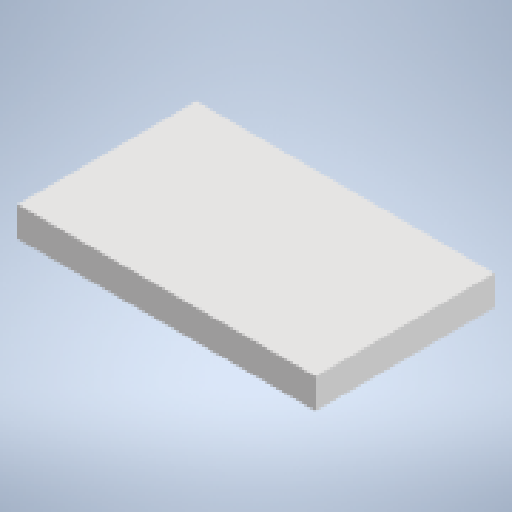
# Autodesk Inventor part: ceiling
Saved by Autodesk Inventor 2024 (Build 280153000, 153)
## iProperties
Created: 2023-05-24
Part Number: ceiling
Material: Generic
Document SubType Name: Modeling
Designer: Patrick
Density: 1 g/cm^3
Appearance: Default
Author: Patrick
Autodesk Inventor part; units mm, degrees
ref_plane "YZ Plane" through (0, 0, 0) normal (1, 0, 0) x (0, 1, 0)
ref_plane "XZ Plane" through (0, 0, 0) normal (0, 1, 0) x (-1, 0, 0)
ref_plane "XY Plane" through (0, 0, 0) normal (0, 0, 1) x (1, 0, 0)
sketch "Sketch1" plane through (0, 0, 0) normal (0, 1, 0) x (-1, 0, 0)
  line L0 (-500, -300) -> (500, -300)
  line L1 (500, -300) -> (500, 300)
  line L2 (500, 300) -> (-500, 300)
  line L3 (-500, 300) -> (-500, -300)
  line L4 (-500, -300) -> (500, 300) construction
  line L5 (500, -300) -> (-500, 300) construction
  point P0 (0, 0)
  dimension "d0" = 1000
  dimension "d1" = 600
  constraints: 12 end point, 2 midpoint, 2 parallel, 1 horizontal, 1 perpendicular
  measures "d0" distance of L2.end L1.end
  measures "d1" distance of L1.end L0.end
extrude "Extrusion1" add sketch "Sketch1" against normal blind 100
body "Solid1"
